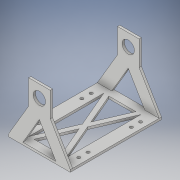
# Autodesk Inventor part: Square Support
Saved by Autodesk Inventor 2019 (Build 230136000, 136)
## iProperties
Created: 2019-04-16
Part Number: Square Support
Material: Generic
Document SubType Name: Modeling
Designer: kyle.fuchs
Density: 1 g/cm^3
Appearance: Default
Author: kyle.fuchs
Autodesk Inventor part; units mm, degrees
ref_plane "YZ Plane" through (0, 0, 0) normal (1, 0, 0) x (0, 1, 0)
ref_plane "XZ Plane" through (0, 0, 0) normal (0, 1, 0) x (-1, 0, 0)
sketch "Sketch1" plane through (0, 0, 0) normal (0, 1, 0) x (-1, 0, 0)
  line L0 (-127, 228.6) -> (-127, -228.6)
  line L1 (-65.8371, -177.8) -> (65.8371, -177.8)
  line L2 (127, -228.6) -> (127, 228.6)
  line L3 (65.8371, 177.8) -> (-65.8371, 177.8)
  line L4 (127, -228.6) -> (-127, -228.6)
  line L5 (-127, 228.6) -> (127, 228.6)
  line L6 (-76.2, 153.6199) -> (-76.2, -153.6199)
  line L7 (76.2, -153.6199) -> (76.2, 153.6199)
  line L8 (76.2, -153.6199) -> (10.3629, 0)
  line L9 (0, 24.1801) -> (-65.8371, 177.8)
  line L10 (65.8371, -177.8) -> (0, -24.1801)
  line L11 (-10.3629, 0) -> (-76.2, 153.6199)
  line L12 (76.2, 153.6199) -> (10.3629, 0)
  line L13 (0, -24.1801) -> (-65.8371, -177.8)
  line L14 (65.8371, 177.8) -> (0, 24.1801)
  line L15 (-10.3629, 0) -> (-76.2, -153.6199)
  point P0 (0, 0)
  point P1 (-127, 155.9501)
  point P2 (127, -155.9501)
  point P3 (-127, -155.9501)
  point P4 (127, 155.9501)
  constraints: 32 end point, 4 point on line, 2 parallel, 2 perpendicular, 1 vertical
extrude "Extrusion3" add sketch "Sketch1" along normal blind 9.525
sketch "Sketch7" plane through (0, 9.525, 0) normal (0, 1, 0) x (1, 0, 0)
  line L0 (0, 24.1801) -> (-65.8371, 177.8) projected
  line L1 (-127, 228.6) -> (-127, -228.6) projected
  line L2 (-76.2, 153.6199) -> (-76.2, -153.6199) projected
  circle A0 centre (-101.6, 127) radius 6.35
  circle A1 centre (-101.6, 88.9) radius 6.35
  line L3 (127, 228.6) -> (-127, 228.6) projected
  line L4 (-127, -228.6) -> (127, -228.6) projected
  circle A2 centre (101.6, 127) radius 6.35
  circle A3 centre (101.6, 88.9) radius 6.35
  line L5 (127, -228.6) -> (127, 228.6) projected
  circle A4 centre (-101.6, -127) radius 6.35
  circle A5 centre (-101.6, -88.9) radius 6.35
  circle A6 centre (101.6, -127) radius 6.35
  circle A7 centre (101.6, -88.9) radius 6.35
  point P0 (0, 0)
  constraints: 8 centre point
extrude "Extrusion4" cut sketch "Sketch7" against normal up to next contours A0 | A1 | A2 | A3 | A4 | A5 | A6 | A7
sketch "Sketch8" plane through (127, 0, -228.6) normal (0, 0, -1) x (-1, 0, 0)
  point P0 (127, 0)
ref_plane "Work Plane2" through (0, 0, 177.8) normal (0, 0, 1) x (1, 0, 0)
mirror "Mirror3" about plane through (0, 0, 0) normal (0, 0, 1)
sketch "Sketch13" plane through (0, 0, 177.8) normal (0, 0, 1) x (1, 0, 0)
  line L0 (0, 0) -> (0, 9.525) projected
  line L1 (-127, 9.525) -> (127, 9.525) projected
  line L2 (0, 9.525) -> (-44.45, 9.525)
  line L3 (-44.45, 250.825) -> (44.45, 250.825)
  circle A0 centre (0, 200.025) radius 25.4
  line L4 (-127, 0) -> (-127, 9.525) projected
  line L5 (-44.45, 149.225) -> (-127, 9.525)
  line L6 (127, 0) -> (127, 9.525) projected
  line L7 (44.45, 149.225) -> (127, 9.525)
  line L8 (67.9938, 9.525) -> (0, 124.5914)
  line L9 (0, 124.5914) -> (-67.9938, 9.525)
  line L10 (44.45, 250.825) -> (44.45, 149.225)
  line L11 (-44.45, 149.225) -> (-44.45, 250.825)
  dimension "d52" = 88.9
  dimension "d56" = 50.8
  dimension "d57" = 50.8
  constraints: 16 end point, 3 perpendicular, 3 point on line, 1 centre point, 1 parallel
  measures "d52" distance of L3.start L3.end
  measures "d56" distance between parallel lines of L7 L8
  measures "d57" distance between parallel lines of L5 L9
extrude "Extrusion8" add sketch "Sketch13" along normal blind 9.525 contours L5 L11 L3 L10 L7 L1 L8 L9
mirror "Mirror4" about plane through (0, 0, 0) normal (0, 0, 1) of "Extrusion8"
sketch "Sketch14" plane through (0, 9.525, 0) normal (0, 1, 0) x (1, 0, 0)
  line L0 (-127, 228.6) -> (-127, 187.325) projected
  line L1 (67.9938, 187.325) -> (127, 187.325) projected
  line L2 (-127, 228.6) -> (127, 228.6)
  line L3 (127, 228.6) -> (127, 187.325)
  line L4 (127, 187.325) -> (-127, 187.325)
  line L5 (-127, 187.325) -> (-127, 228.6)
  line L6 (-44.45, -187.325) -> (-127, -187.325) projected
  line L7 (-127, -228.6) -> (127, -228.6) projected
  line L8 (-127, -187.325) -> (127, -187.325)
  line L9 (127, -187.325) -> (127, -228.6)
  line L10 (127, -228.6) -> (-127, -228.6)
  line L11 (-127, -228.6) -> (-127, -187.325)
  point P0 (0, 0)
  constraints: 16 end point, 4 parallel, 2 horizontal, 2 perpendicular
extrude "Extrusion9" cut sketch "Sketch14" against normal blind 25.4
sketch "Sketch15" plane through (0, 9.525, 0) normal (0, 1, 0) x (1, 0, 0)
  line L0 (-76.2, 153.6199) -> (-10.3629, 0) projected
  line L1 (-76.2, 153.6199) -> (76.2, 153.6199)
  line L2 (76.2, 153.6199) -> (76.2, 177.8)
  line L3 (127, 177.8) -> (44.45, 177.8) projected
  line L4 (-76.2, 153.6199) -> (-76.2, 177.8)
  line L5 (-76.2, 177.8) -> (76.2, 177.8)
  line L6 (-44.45, -177.8) -> (-127, -177.8) projected
  line L7 (-76.2, -177.8) -> (76.2, -177.8)
  line L8 (76.2, -177.8) -> (76.2, -152.9852)
  line L9 (76.2, -152.9852) -> (-76.2, -152.9852)
  line L10 (-76.2, -152.9852) -> (-76.2, -177.8)
  point P0 (0, 0)
  constraints: 16 end point, 6 point on line, 4 perpendicular, 1 collinear, 1 horizontal, 1 vertical
extrude "Extrusion10" add sketch "Sketch15" against normal blind 9.525 contours L4 L5 L3 L2 L1
sketch "Sketch16" plane through (0, 9.525, 0) normal (0, 1, 0) x (1, 0, 0)
  line L0 (-76.2, -153.6199) -> (-10.3629, 0) projected
  line L1 (-76.2, -153.6199) -> (-76.2, -177.8)
  line L2 (-127, -177.8) -> (-67.9938, -177.8) projected
  line L3 (76.2, -153.6199) -> (76.2, 153.6199) projected
  line L4 (76.2, -153.6199) -> (-76.2, -153.6199)
  line L5 (-76.2, -153.6199) -> (-76.2, -177.8)
  line L6 (-76.2, -177.8) -> (76.2, -177.8)
  line L7 (76.2, -177.8) -> (76.2, -153.6199)
  point P0 (0, 0)
  constraints: 10 end point, 2 parallel, 1 horizontal, 1 perpendicular, 1 point on line, 1 vertical
extrude "Extrusion11" add sketch "Sketch16" against normal blind 9.525
ref_plane "Work Plane3" through (0, 0, 0) normal (0, 0, 1) x (1, 0, 0)
body "Solid2"
